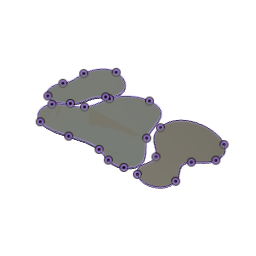
Splat maps v2 (Autodesk Fusion 360 design; units mm, degrees)
Autodesk Fusion 360 part; units mm, degrees
sketch "Sketch1" plane through (0, 0, 0) normal (0, 1, 0) x (1, 0, 0)
  spline S0 degree 3 poles (39.0438, -2.1846) (7.4993, 9.6343) (-8.8559, -29.0224) (4.9183, -57.6125) knots 0 0 0 0 1 1 1 1
  spline S1 degree 3 poles (4.9183, -57.6125) (12.8672, -74.1111) (34.1463, -76.6252) (51.7496, -69.3047) knots 0 0 0 0 1 1 1 1
  spline S2 degree 3 poles (51.7496, -69.3047) (64.4813, -64.009) (74.2921, -52.9318) (88.8971, -54.9679) knots 0 0 0 0 1 1 1 1
  spline S3 degree 3 poles (88.8971, -54.9679) (103.7365, -57.0367) (120.7923, -46.0706) (120.0462, -30.6765) knots 0 0 0 0 1 1 1 1
  spline S4 degree 3 poles (120.0462, -30.6765) (119.3848, -16.9975) (113.1652, -7.8573) (94.2134, -2.1843) knots 0 0 0 0 1 1 1 1
  spline S5 degree 3 poles (94.2134, -2.1843) (68.1614, 5.6143) (67.5047, -12.847) (39.0438, -2.1846) knots 0 0 0 0 1 1 1 1
extrude "Extrude1" add sketch "Sketch1" along normal blind 3 makes body 1
sketch "Sketch2" plane through (0, 0, 0) normal (0, 1, 0) x (1, 0, 0)
  spline S0 degree 3 poles (52.7795, 131.444) (16.8166, 127.5631) (13.1086, 101.8442) (-13.6442, 82.8007) knots 0 0 0 0 1 1 1 1
  spline S1 degree 3 poles (-13.6442, 82.8007) (-31.231, 70.282) (-49.2282, 97.4864) (-70.2425, 73.2078) knots 0 0 0 0 1 1 1 1
  spline S2 degree 3 poles (-70.2425, 73.2078) (-91.3359, 49.3029) (-81.3456, 5.2151) (-43.9252, 13.7184) knots 0 0 0 0 1 1 1 1
  spline S3 degree 3 poles (-43.9252, 13.7184) (-24.3337, 16.1737) (-6.0765, 48.5766) (13.2408, 30.0963) knots 0 0 0 0 1 1 1 1
  spline S4 degree 3 poles (13.2408, 30.0963) (22.1841, 20.1607) (28.6805, 5.5877) (43.4448, 3.6217) knots 0 0 0 0 1 1 1 1
  spline S5 degree 3 poles (43.4448, 3.6217) (62.9673, 0.869) (74.2776, 7.6526) (85.201, 22.7163) knots 0 0 0 0 1 1 1 1
  spline S6 degree 3 poles (85.201, 22.7163) (112.7314, 60.6834) (110.2407, 139.0052) (52.7795, 131.444) knots 0 0 0 0 1 1 1 1
extrude "Extrude2" add sketch "Sketch2" along normal blind 3 separate body makes body 2
sketch "Sketch3" plane through (0, 3, 0) normal (0, 1, 0) x (-1, 0, 0)
  spline S0 degree 3 poles (-94.2134, 2.1843) (-68.1614, -5.6143) (-67.5047, 12.847) (-39.0438, 2.1846) knots 0 0 0 0 1 1 1 1
  spline S1 degree 3 poles (-39.0438, 2.1846) (-7.4993, -9.6343) (8.8559, 29.0224) (-4.9183, 57.6125) knots 0 0 0 0 1 1 1 1
  spline S2 degree 3 poles (-4.9183, 57.6125) (-12.8672, 74.1111) (-34.1463, 76.6252) (-51.7496, 69.3047) knots 0 0 0 0 1 1 1 1
  spline S3 degree 3 poles (-51.7496, 69.3047) (-64.4813, 64.009) (-74.2921, 52.9318) (-88.8971, 54.9679) knots 0 0 0 0 1 1 1 1
  spline S4 degree 3 poles (-88.8971, 54.9679) (-103.7365, 57.0367) (-120.7923, 46.0706) (-120.0462, 30.6765) knots 0 0 0 0 1 1 1 1
  spline S5 degree 3 poles (-120.0462, 30.6765) (-119.3848, 16.9975) (-113.1652, 7.8573) (-94.2134, 2.1843) knots 0 0 0 0 1 1 1 1
  line L0 (207.4715, -175.1349) -> (-275.1285, -175.1349)
  line L1 (-275.1285, -175.1349) -> (-275.1285, 104.2651)
  line L2 (-275.1285, 104.2651) -> (207.4715, 104.2651)
  line L3 (207.4715, 104.2651) -> (207.4715, -175.1349)
  dimension "d5" = 482.6
  dimension "d6" = 279.4
  constraint horizontal L0
  constraint vertical L1
  constraint horizontal L2
  constraint vertical L3
  measures "d5" distance of L0.start L0.end
  measures "d6" distance of L0.start L2.end
move_body "Move1" bodies 1 to x (0.802665, 0, -0.59643) y (0, 1, 0) z (0.59643, 0, 0.802665) at (129.4105, 0, 35.121)
scale "Scale1" factor 1.51739 about (162.0525, 3, 13.5877) bodies 1
move_body "Move2" bodies 1 to x (1, 0, 0) y (0, 1, 0) z (0, 0, 1) at (-33.63, 0, -24.3171)
scale "Scale2" factor 1.77608 about (-13.6442, 0, -82.8007) bodies 2
move_body "Move3" bodies 1 to x (0.998162, 0, 0.060604) y (0, 1, 0) z (-0.060604, 0, 0.998162) at (-4.1512, 0, -4.9366)
move_body "Move4" bodies 2 to x (-1, 0, 0) y (0, 1, 0) z (0, 0, -1) at (130.3811, 0, -146.9374)
sketch "Sketch4" plane through (0, 0, 0) normal (0, 1, 0) x (1, 0, 0)
  spline S0 degree 3 poles (-120.5307, -99.8397) (-137.1386, -103.8878) (-154.3796, -96.2314) (-167.6238, -86.0295) knots 0 0 0 0 1 1 1 1
  spline S1 degree 3 poles (-167.6238, -86.0295) (-180.8673, -75.8275) (-191.8097, -62.9499) (-205.8524, -53.7816) knots 0 0 0 0 1 1 1 1
  spline S2 degree 3 poles (-205.8524, -53.7816) (-231.6887, -36.9152) (-264.6354, -34.5358) (-295.8661, -31.5903) knots 0 0 0 0 1 1 1 1
  spline S3 degree 3 poles (-295.8661, -31.5903) (-327.0974, -28.6454) (-360.3055, -23.7241) (-383.3214, -3.4479) knots 0 0 0 0 1 1 1 1
  spline S4 degree 3 poles (-383.3214, -3.4479) (-406.3392, 16.8284) (-411.857, 57.7195) (-386.3273, 75.6644) knots 0 0 0 0 1 1 1 1
  spline S5 degree 3 poles (-386.3273, 75.6644) (-364.4219, 91.0618) (-332.128, 82.8475) (-308.9769, 96.4328) knots 0 0 0 0 1 1 1 1
  spline S6 degree 3 poles (-308.9769, 96.4328) (-288.4467, 108.4784) (-281.4487, 133.5005) (-267.0869, 152.0657) knots 0 0 0 0 1 1 1 1
  spline S7 degree 3 poles (-267.0869, 152.0657) (-246.1624, 179.1154) (-206.8406, 191.5732) (-173.7101, 181.6506) knots 0 0 0 0 1 1 1 1
  spline S8 degree 3 poles (-173.7101, 181.6506) (-96.6291, 158.5655) (-129.2182, 90.454) (-118.2795, 35.46) knots 0 0 0 0 1 1 1 1
  spline S9 degree 3 poles (-118.2795, 35.46) (-111.1937, -0.1681) (-51.5951, -83.0378) (-120.5307, -99.8397) knots 0 0 0 0 1 1 1 1
extrude "Extrude3" add sketch "Sketch4" along normal blind 3 separate body makes body 3
scale "Scale3" factor 0.927669 about (-205.8524, 0, 53.7816) bodies 3
move_body "Move5" bodies 3 to x (0.928886, 0, -0.370365) y (0, 1, 0) z (0.370365, 0, 0.928886) at (221.042, 0, -57.7848)
move_body "Move6" bodies 1 to x (-0.869383, 0, 0.494138) y (0, 1, 0) z (-0.494138, 0, -0.869383) at (19.6704, 0, -155.5305)
move_body "Move7" bodies 2 to x (0.312738, 0, 0.94984) y (0, 1, 0) z (-0.94984, 0, 0.312738) at (92.9439, 0, -116.9775)
scale "Scale4" factor 0.783006 about (245.3644, 5.3282, -200.3592) bodies 2
move_body "Move8" bodies 2 to x (0.968165, 0, 0.250314) y (0, 1, 0) z (-0.250314, 0, 0.968165) at (-52.1675, 0, -11.5945)
move_body "Move9" bodies 1 to x (1, 0, 0) y (0, 1, 0) z (0, 0, 1) at (0, 1.5, 0)
extrude "Extrude4" cut 1 faces at (183.2378, 5.3282, -77.8057) along direction (0, -1, 0) blind 1.172 on bodies 2 bodies 2
extrude "Extrude5" add 1 faces at (5.565, 2.783, -10.4932) along direction (0, 1, 0) blind 0.217 on bodies 3 bodies 3
extrude "Extrude6" cut 1 faces at (-128.5808, 4.5, -125.2968) along direction (0, -1, 0) blind 1.552 on bodies 1 bodies 1
sketch "Sketch5" plane through (0, 3, 0) normal (0, 1, 0) x (-1, 0, 0)
  spline S0 degree 3 poles (-94.5476, -38.5747) (-66.2271, -82.2047) (-70.9076, -152.0931) (3.4445, -145.5023) knots -1 -1 -1 -1 0 0 0 0
  spline S1 degree 3 poles (3.4445, -145.5023) (35.4023, -142.6698) (65.0055, -118.4249) (73.7425, -87.927) knots -1 -1 -1 -1 0 0 0 0
  spline S2 degree 3 poles (73.7425, -87.927) (79.7395, -66.995) (77.1727, -43.0292) (90.725, -25.5958) knots -1 -1 -1 -1 0 0 0 0
  spline S3 degree 3 poles (90.725, -25.5958) (106.0067, -5.9352) (136.6565, -1.918) (150.2422, 18.8761) knots -1 -1 -1 -1 0 0 0 0
  spline S4 degree 3 poles (150.2422, 18.8761) (166.0757, 43.1106) (147.2718, 76.4506) (120.4709, 86.0143) knots -1 -1 -1 -1 0 0 0 0
  spline S5 degree 3 poles (120.4709, 86.0143) (93.6717, 95.5786) (63.3655, 88.4097) (35.4417, 80.217) knots -1 -1 -1 -1 0 0 0 0
  spline S6 degree 3 poles (35.4417, 80.217) (7.5183, 72.025) (-21.6894, 62.7557) (-49.7473, 68.4127) knots -1 -1 -1 -1 0 0 0 0
  spline S7 degree 3 poles (-49.7473, 68.4127) (-64.998, 71.4882) (-78.8515, 78.8253) (-93.7686, 83.0662) knots -1 -1 -1 -1 0 0 0 0
  spline S8 degree 3 poles (-93.7686, 83.0662) (-108.6862, 87.3068) (-126.1733, 87.9807) (-139.0935, 78.7864) knots -1 -1 -1 -1 0 0 0 0
  spline S9 degree 3 poles (-139.0935, 78.7864) (-192.7225, 40.6236) (-112.8944, -10.3085) (-94.5476, -38.5747) knots -1 -1 -1 -1 0 0 0 0
  spline S10 degree 3 poles (84.8435, -87.0823) (93.648, -79.0944) (98.5464, -72.2675) (104.403, -59.7717) (105.3559, -54.0949) (107.0462, -43.1858) (107.7935, -37.9623) (112.2411, -26.4207) (116.0534, -20.0486) (123.1695, -12.657) knots -12.448534 -12.448534 -12.448534 -12.448534 -9.249279 -9.249279 -6.044044 -6.044044 -3.078102 -3.078102 0 0 0 0
  spline S11 degree 3 poles (135.9101, -171.624) (129.0656, -171.442) (122.2637, -170.2932) (109.422, -166.3295) (103.3466, -163.5703) (91.0593, -155.9238) (84.9457, -150.6551) (76.5995, -139.9529) (73.7361, -134.9071) (70.5, -125.0503) (69.7954, -120.4483) (70.2296, -110.924) (71.4403, -106.2536) (76.2177, -96.1991) (80.2015, -91.2933) (84.8435, -87.0823) knots -12.840308 -12.840308 -12.840308 -12.840308 -10.796898 -10.796898 -8.82626 -8.82626 -6.468883 -6.468883 -4.750054 -4.750054 -3.34686 -3.34686 -1.880244 -1.880244 0 0 0 0
  spline S12 degree 3 poles (184.2168, -116.5701) (183.7892, -121.8087) (182.8355, -127.0321) (179.938, -136.9815) (178.0059, -141.7722) (172.5319, -151.7834) (168.6823, -156.9032) (160.1963, -164.4744) (155.9142, -167.1953) (146.2841, -170.9191) (141.1613, -171.7636) (135.9101, -171.624) knots -8.094249 -8.094249 -8.094249 -8.094249 -6.52078 -6.52078 -4.990726 -4.990726 -3.100758 -3.100758 -1.575924 -1.575924 0 0 0 0
  spline S13 degree 3 poles (190.6826, -56.4975) (188.8834, -59.0496) (187.417, -61.7617) (185.2124, -67.4156) (184.476, -70.2323) (183.0476, -78.8663) (183.1258, -84.7518) (183.9327, -99.2224) (184.9236, -107.9027) (184.2168, -116.5701) knots -6.358772 -6.358772 -6.358772 -6.358772 -5.371603 -5.371603 -4.442064 -4.442064 -2.608865 -2.608865 0 0 0 0
  spline S14 degree 3 poles (179.5522, 2.3986) (182.5421, 1.0378) (185.2555, -0.775) (189.9638, -5.1991) (191.9066, -7.7157) (196.0097, -14.9108) (197.5404, -19.8888) (198.9466, -30.8785) (198.5166, -37.0131) (195.6931, -47.6729) (193.5935, -52.3685) (190.6826, -56.4975) knots -6.782902 -6.782902 -6.782902 -6.782902 -5.796102 -5.796102 -4.840875 -4.840875 -3.306222 -3.306222 -1.515598 -1.515598 0 0 0 0
  spline S15 degree 3 poles (123.1695, -12.657) (127.1418, -8.5307) (131.5478, -4.5094) (140.0526, 1.4424) (144.1566, 3.7075) (153.1465, 6.7582) (157.802, 7.3907) (168.251, 6.666) (173.8268, 5.0052) (179.5522, 2.3986) knots -7.018167 -7.018167 -7.018167 -7.018167 -5.08013 -5.08013 -3.51787 -3.51787 -1.887232 -1.887232 0 0 0 0
  spline S16 degree 3 poles (-87.5844, -89.3328) (-86.5582, -94.5037) (-85.9834, -99.7835) (-86.1187, -109.6914) (-86.6827, -114.2917) (-89.534, -125.1376) (-92.366, -130.9684) (-100.9005, -142.1226) (-106.6638, -146.9046) (-122.147, -155.9759) (-132.8883, -159.52) (-162.073, -164.2514) (-181.4406, -163.2849) (-212.0689, -155.88) (-224.6286, -151.0322) (-235.5383, -144.1572) knots -21.506737 -21.506737 -21.506737 -21.506737 -19.655359 -19.655359 -18.02616 -18.02616 -15.715213 -15.715213 -13.088916 -13.088916 -9.410611 -9.410611 -3.868571 -3.868571 0 0 0 0
  spline S17 degree 3 poles (-161.0951, -1.5527) (-146.1832, -19.8542) (-129.3708, -29.4367) (-108.9918, -46.705) (-103.181, -52.6065) (-93.522, -67.7263) (-89.7203, -77.0787) (-87.5844, -89.3328) knots -15.237215 -15.237215 -15.237215 -15.237215 -7.34642 -7.34642 -3.731665 -3.731665 0 0 0 0
  spline S18 degree 3 poles (-179.5256, 76.1234) (-174.5658, 72.3656) (-171.0037, 68.6083) (-166.1622, 61.3673) (-164.562, 57.6498) (-162.335, 46.679) (-163.3195, 39.8596) (-165.5905, 27.6111) (-166.7993, 22.1404) (-167.0633, 13.5932) (-166.7841, 10.45) (-164.8954, 4.0563) (-163.2707, 1.1175) (-161.0951, -1.5527) knots -7.892389 -7.892389 -7.892389 -7.892389 -6.64571 -6.64571 -5.504306 -5.504306 -3.588687 -3.588687 -1.993039 -1.993039 -1.033312 -1.033312 0 0 0 0
  spline S19 degree 3 poles (-259.7015, 34.2225) (-261.1093, 38.9657) (-262.0064, 43.8875) (-262.1791, 53.0568) (-261.6687, 57.2456) (-259.0573, 65.7234) (-256.8645, 69.7721) (-250.5792, 77.3147) (-246.4599, 80.4966) (-235.8985, 86.0494) (-229.21, 87.8462) (-214.6215, 89.1954) (-206.5904, 88.354) (-191.9846, 83.9722) (-185.3498, 80.6244) (-179.5256, 76.1234) knots -12.367571 -12.367571 -12.367571 -12.367571 -10.874168 -10.874168 -9.596807 -9.596807 -8.19125 -8.19125 -6.624496 -6.624496 -4.581714 -4.581714 -2.208226 -2.208226 0 0 0 0
  spline S20 degree 3 poles (-231.804, -43.6279) (-229.693, -41.1124) (-227.8637, -38.3245) (-225.6087, -32.6801) (-225.0526, -30.0032) (-225.0056, -23.9087) (-225.731, -20.7123) (-230.1153, -9.3696) (-236.8768, -1.3835) (-248.1415, 12.3957) (-252.7083, 18.1242) (-257.6083, 27.2205) (-259.0138, 30.6415) (-259.7015, 34.2225) knots -9.010068 -9.010068 -9.010068 -9.010068 -7.945624 -7.945624 -7.042989 -7.042989 -5.974759 -5.974759 -3.107241 -3.107241 -1.093941 -1.093941 0 0 0 0
  spline S21 degree 3 poles (-265.8124, -87.9372) (-265.6451, -85.4543) (-265.2081, -83.0273) (-263.7965, -78.3875) (-262.8714, -76.2365) (-259.4701, -70.0358) (-256.4459, -66.3778) (-246.4474, -56.1933) (-238.2945, -50.2836) (-231.804, -43.6279) knots -5.568648 -5.568648 -5.568648 -5.568648 -4.84481 -4.84481 -4.158562 -4.158562 -2.788957 -2.788957 0 0 0 0
  spline S22 degree 3 poles (-235.5383, -144.1572) (-243.6355, -139.0543) (-250.16, -133.7795) (-258.9894, -122.9782) (-261.8498, -117.7512) (-265.772, -104.9999) (-266.5076, -97.1872) (-265.8124, -87.9372) knots -8.211574 -8.211574 -8.211574 -8.211574 -5.19353 -5.19353 -2.782841 -2.782841 0 0 0 0
